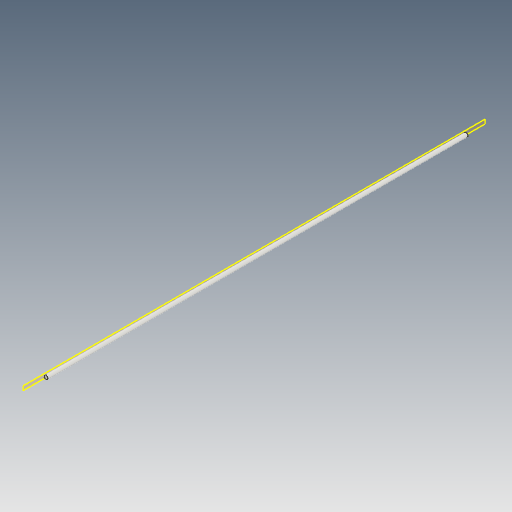
# Autodesk Inventor part: Tubo-2_1_8
Saved by Autodesk Inventor 2021 (Build 250183000, 183)
## iProperties
Created: 2021-04-30
Part Number: Tubo-2_1_8
Material: Steel AISI 1050
Document SubType Name: Modeling
Designer: Nelson
Density: 7.85 g/cm^3
Appearance: Steel
Author: Nelson
Autodesk Inventor part; units mm, degrees
ref_plane "XZ Plane" through (0, 0, 0) normal (0, 1, 0) x (-1, 0, 0)
ref_plane "XY Plane" through (0, 0, 0) normal (0, 0, 1) x (1, 0, 0)
sketch "Sketch1" plane through (0, 0, 0) normal (0, 0, 1) x (1, 0, 0)
  circle A0 centre (0, 0) radius 26.9875
  dimension "d0" = 53.975
  constraints: 1 centre point, 1 coincident
  measures "d0" diameter of A0
extrude "Extrusion1" add sketch "Sketch1" against normal blind 6000
ref_plane "Work Plane1" through (-26.9875, 0, 0) normal (1, 0, 0) x (0, 1, 0)
body "Solid1"
